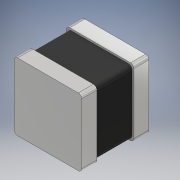
# Autodesk Inventor part: Moteur pas à pas
Saved by Autodesk Inventor 2017 (Build 210142000, 142)
## iProperties
Part Number: Moteur pas à pas
Material: Générique
Document SubType Name: Modeling
Designer: sasha
Density: 1 g/cm^3
Appearance: Par défaut
Author: sasha
Autodesk Inventor part; units mm, degrees
ref_plane "YZ Plane" through (0, 0, 0) normal (1, 0, 0) x (0, 1, 0)
ref_plane "XZ Plane" through (0, 0, 0) normal (0, 1, 0) x (-1, 0, 0)
ref_plane "XY Plane" through (0, 0, 0) normal (0, 0, 1) x (1, 0, 0)
sketch "Esquisse1" plane through (0, 0, 0) normal (0, 1, 0) x (-1, 0, 0)
  line L0 (40, 0) -> (0, 0)
  line L1 (0, 0) -> (0, -40)
  line L2 (0, -40) -> (40, -40)
  line L3 (40, -40) -> (40, 0)
  dimension "d0" = 40
  dimension "d1" = 40
  constraints: 8 end point, 2 parallel, 1 coincident, 1 horizontal, 1 perpendicular
  measures "d0" distance of L1.end L2.end
  measures "d1" distance of L2.end L0.start
extrude "Extrusion1" add sketch "Esquisse1" along normal blind 9
sketch "Esquisse2" plane through (0, 9, 0) normal (0, 1, 0) x (1, 0, 0)
  line L0 (-39, 1) -> (-1, 1)
  line L1 (-1, 1) -> (-1, 39)
  line L2 (-1, 39) -> (-39, 39)
  line L3 (-39, 39) -> (-39, 1)
  line L4 (-40, 40) -> (-40, 0) projected
  line L5 (0, 0) -> (0, 40) projected
  line L6 (0, 40) -> (-40, 40) projected
  line L7 (-40, 0) -> (0, 0) projected
  dimension "d4" = 1
  dimension "d5" = 1
  dimension "d6" = 1
  dimension "d7" = 1
  constraints: 8 end point, 2 parallel, 1 horizontal, 1 perpendicular
  measures "d4" distance between parallel lines of L4 L3
  measures "d5" distance between parallel lines of L5 L1
  measures "d6" distance between parallel lines of L6 L2
  measures "d7" distance between parallel lines of L7 L0
extrude "Extrusion2" add sketch "Esquisse2" along normal blind 22 contours L3 L2 L1 L0
sketch "Esquisse3" plane through (0, 31, 0) normal (0, 1, 0) x (1, 0, 0)
  line L0 (0, 0) -> (0, 40) projected
  line L1 (0, 0) -> (-40.0621, 0)
  line L2 (-40.0621, 0) -> (-40.0621, 40)
  line L3 (-40.0621, 40) -> (0, 40)
  line L4 (0, 40) -> (0, 0)
  constraints: 8 end point, 2 parallel, 1 horizontal, 1 perpendicular
extrude "Extrusion3" add sketch "Esquisse3" along normal blind 9
fillet "Congé1" radius 2 12 edges at (-40, 4.5, -40) (-40, 4.5, 0) (-40.0621, 35.5, 0) (-40.0621, 35.5, -40) (-39, 20, -39) (-39, 20, -1) (0, 4.5, 0) (0, 4.5, -40) (0, 35.5, -40) (0, 35.5, 0) (-1, 20, -1) (-1, 20, -39)
sketch "Esquisse4" plane through (0, 40, 0) normal (0, 1, 0) x (1, 0, 0)
  line L0 (-38.0621, 0) -> (-2, 0) projected
  line L1 (-20.031, 0) -> (-20.031, 40) construction
  line L2 (-2, 40) -> (-38.0621, 40) projected
  line L3 (0, 2) -> (0, 38) projected
  line L4 (0, 20) -> (-40, 20)
  line L5 (-40, 38) -> (-40, 2) projected
  circle A0 centre (-20, 20) radius 12.5
  circle A1 centre (-20, 20) radius 1
  point P0 (0, 0)
  dimension "d13" = 25
  dimension "d14" = 2
  constraints: 5 midpoint, 4 end point, 2 centre point, 1 coincident
  measures "d13" diameter of A0
  measures "d14" diameter of A1
extrude "Extrusion4" add sketch "Esquisse4" along normal blind 3 contours A0 L4 A1 | L4 A1 A0
sketch "Esquisse5" plane through (0, 40, 0) normal (0, 1, 0) x (1, 0, 0)
  circle A0 centre (-20, 20) radius 1 projected
  circle A1 centre (-20, 20) radius 1
  point P0 (0, 0)
  constraints: 2 coincident, 1 centre point
extrude "Extrusion5" add sketch "Esquisse5" along normal blind 10
